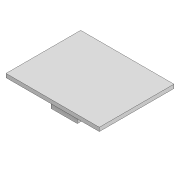
# Autodesk Inventor part: Moving platform
Saved by Autodesk Inventor 2020 (Build 240168000, 168)
## iProperties
Created: 2020-08-18
Part Number: Moving platform
Material: Generic
Document SubType Name: Modeling
Designer: ferrerx
Density: 1 g/cm^3
Appearance: Anodized - Black
Mass: 1.44418 g
Surface Area: 16.2651 cm^2
Volume: 1.44418 cm^3
Author: ferrerx
Autodesk Inventor part; units mm, degrees
ref_plane "YZ Plane" through (0, 0, 0) normal (1, 0, 0) x (0, 1, 0)
ref_plane "XZ Plane" through (0, 0, 0) normal (0, 1, 0) x (-1, 0, 0)
sketch "Sketch1" plane through (0, 0, 0) normal (0, 1, 0) x (-1, 0, 0)
  line L0 (0, 0) -> (25, 0)
  line L1 (25, 0) -> (25, -13.8)
  line L2 (25, -13.8) -> (0, -13.8)
  line L3 (0, -13.8) -> (0, 0)
  dimension "d0" = 25
  dimension "d1" = 13.8
  constraints: 8 end point, 2 parallel, 1 horizontal, 1 perpendicular
  measures "d0" distance of L1.end L2.end
  measures "d1" distance of L2.end L0.start
extrude "Extrusion1" add sketch "Sketch1" along normal blind 4.2
sketch "Sketch2" plane through (0, 0, 0) normal (1, 0, 0) x (0, 0, -1)
  line L0 (0, 0) -> (0, 4.2)
  line L1 (0, 2) -> (13.8, 2)
  line L2 (13.8, 0) -> (13.8, 4.2)
  circle A0 centre (2.4, 2) radius 1.05
  circle A1 centre (11.4, 2) radius 1.05
  line L3 (0, 0) -> (13.8, 0) projected
  line L4 (6.9, 0) -> (6.9, 2.0025)
  line L5 (0, 4.2) -> (13.8, 4.2) projected
  dimension "d4" = 9
  dimension "d7" = 4.5
  dimension "d15" = 2.2
  constraints: 8 end point, 3 point on line, 2 centre point, 1 midpoint, 1 vertical
  measures "d4" distance of A1.centre A0.centre
  measures "d7" distance from line of L4 A0.centre
  measures "d15" distance between parallel lines of L5 L1
extrude "Extrusion2" cut sketch "Sketch2" against normal blind 20 contours A0 L1 | L1 A0 | A1 L1 | L1 A1
sketch "Sketch3" plane through (0, 4.2, 0) normal (0, 1, 0) x (1, 0, 0)
  line L0 (0, 6.9) -> (-25, 6.9)
  line L1 (0, -3.1) -> (-25, -3.1)
  line L2 (-25, -3.1) -> (-25, 16.9)
  line L3 (-25, 16.9) -> (0, 16.9)
  line L4 (0, 16.9) -> (0, -3.1)
  line L5 (0, -3.1) -> (-25, 16.9) construction
  line L6 (-25, -3.1) -> (0, 16.9) construction
  line L7 (-25, 13.8) -> (-25, 0) projected
  line L8 (0, 0) -> (0, 13.8) projected
  line L9 (0, 13.8) -> (-25, 13.8) projected
  point P0 (-12.5, 6.9)
  dimension "d10" = 20
  dimension "d11" = 6.9
  dimension "d12" = 25
  constraints: 14 end point, 5 midpoint, 2 horizontal, 2 parallel, 1 perpendicular
  measures "d10" distance of L3.end L1.start
  measures "d11" distance between parallel lines of L9 L0
  measures "d12" distance of L2.end L3.end
extrude "Extrusion3" add sketch "Sketch3" along normal blind 1
sketch "Sketch4" plane through (0, 5.2, 0) normal (0, 1, 0) x (1, 0, 0)
  circle A0 centre (-21, 12.9) radius 0.25
  line L0 (0, 16.9) -> (-25, 16.9) projected
  line L1 (-25, 16.9) -> (-25, -3.1) projected
  line L2 (-21.25, 12.9) -> (-20.75, 12.9)
  point P0 (0, 0)
  dimension "d16" = 4
  dimension "d17" = 4
  dimension "d18" = 0.5
  constraints: 2 end point, 2 point on circle, 1 centre point, 1 horizontal
  measures "d16" distance from line of L0 A0.centre
  measures "d17" distance from line of L1 A0.centre
  measures "d18" diameter of A0
ref_plane "Work Plane1" through (-21.25, 5.2, -12.9) normal (0, 0, 1) x (1, 0, 0)
sketch "Sketch5" plane through (-21.25, 5.2, -12.9) normal (0, 0, 1) x (1, 0, 0)
  line L0 (-3.75, 0) -> (21.25, 0) projected
  line L1 (0.2469, 0) -> (0.2469, 2)
  line L2 (0.2469, 2) -> (0.9969, 0)
  line L3 (0.9969, 0) -> (0.2469, 0)
  line L4 (21.25, -1) -> (-3.75, -1) projected
  point P0 (21.25, -5.2)
  dimension "d21" = 2
  dimension "d28" = 0.75
  constraints: 6 end point, 1 parallel, 1 point on line, 1 vertical
  measures "d21" distance of L1.start L1.end
  measures "d28" distance of L1.start L2.end
revolve "Revolution1" [suppressed]
pattern_linear "Rectangular Pattern1" [suppressed]
sketch "Sketch6" plane through (0, 0, 0) normal (1, 0, 0) x (0, 0, -1)
  circle A0 centre (2.4, 2) radius 1.05 projected
  circle A1 centre (2.4, 2) radius 1.1
  circle A2 centre (11.4, 2) radius 1.05 projected
  circle A3 centre (11.4, 2) radius 1.1
  point P0 (0, 0)
  dimension "d29" = 2.2
  dimension "d30" = 2.2
  constraints: 2 centre point, 2 coincident
  measures "d29" diameter of A3
  measures "d30" diameter of A1
extrude "Extrusion4" cut sketch "Sketch6" against normal blind 30.5 contours A0 | A1 | A2 | A3
sketch "Sketch7" plane through (0, 5.2, 0) normal (0, 1, 0) x (1, 0, 0)
  line L0 (0, 6.9) -> (-25, 6.9) construction
  line L1 (0, 16.9) -> (-25, 16.9) projected
  line L2 (-13.35, 4.85) -> (-11.65, 4.85)
  line L3 (-11.65, 4.85) -> (-11.65, 8.95)
  line L4 (-11.65, 8.95) -> (-13.35, 8.95)
  line L5 (-13.35, 8.95) -> (-13.35, 4.85)
  line L6 (-13.35, 4.85) -> (-11.65, 8.95) construction
  line L7 (-11.65, 4.85) -> (-13.35, 8.95) construction
  line L8 (0, -3.1) -> (0, 16.9) projected
  point P0 (0, 0)
  point P1 (-12.5, 6.9)
  dimension "d33" = 10
  dimension "d34" = 1.7
  dimension "d35" = 4.1
  dimension "d36" = 11.65
  constraints: 14 end point, 3 midpoint, 2 horizontal, 2 parallel, 1 perpendicular
  measures "d33" distance between parallel lines of L1 L0
  measures "d34" distance of L2.start L2.end
  measures "d35" distance of L2.end L3.end
  measures "d36" distance between parallel lines of L8 L3
extrude "Extrusion5" cut sketch "Sketch7" against normal blind 8.45
sketch "Sketch8" plane through (0, 0, 0) normal (1, 0, 0) x (0, 0, -1)
  circle A0 centre (2.4, 2) radius 1.1 projected
  circle A1 centre (11.4, 2) radius 1.1 projected
  line L0 (2.4, 2) -> (11.4, 2) construction
  circle A2 centre (6.9, 2) radius 1.1
  point P0 (0, 0)
  dimension "d39" = 2.2
  dimension "d40" = 4.5
  constraints: 2 end point, 1 centre point, 1 horizontal, 1 midpoint
  measures "d39" diameter of A2
  measures "d40" distance of L0.start A2.centre
extrude "Extrusion6" cut sketch "Sketch8" against normal blind 31.95 contours A2
sketch "Sketch9" plane through (0, 5.2, 0) normal (0, 1, 0) x (1, 0, 0)
  line L0 (-13.35, 4.85) -> (-13.35, 8.95) projected
  line L1 (-11.65, 4.85) -> (-11.65, 8.95) projected
  line L2 (-13.35, 8.95) -> (-11.65, 8.95)
  line L3 (-11.65, 8.95) -> (-11.65, 4.85)
  line L4 (-11.65, 4.85) -> (-13.35, 4.85)
  line L5 (-13.35, 4.85) -> (-13.35, 8.95)
  point P0 (0, 0)
  constraints: 8 end point, 2 parallel, 1 horizontal, 1 perpendicular
extrude "Extrusion7" add sketch "Sketch9" against normal blind 0.5
sketch "Sketch10" plane through (0, 0, 0) normal (1, 0, 0) x (0, 0, -1)
  line L0 (0, 0) -> (13.8, 0)
  line L1 (13.8, 0) -> (13.8, 4.2)
  line L2 (13.8, 4.2) -> (0, 4.2)
  line L3 (0, 4.2) -> (0, 0)
  line L4 (13.8, 4.2) -> (16.9, 4.2) projected
  line L5 (13.8, 0) -> (13.8, 4.2) projected
  constraints: 8 end point, 2 collinear, 2 parallel, 1 horizontal, 1 perpendicular
extrude "Extrusion8" cut sketch "Sketch10" against normal blind 9
sketch "Sketch11" plane through (-25, 0, -13.8) normal (-1, 0, 0) x (0, 0, 1)
  line L0 (13.8, 0) -> (13.8, 4.2) projected
  line L1 (0, 0) -> (13.8, 0)
  line L2 (13.8, 0) -> (13.8, 4.2)
  line L3 (13.8, 4.2) -> (0, 4.2)
  line L4 (0, 4.2) -> (0, 0)
  line L5 (13.8, 4.2) -> (16.9, 4.2) projected
  constraints: 8 end point, 2 parallel, 1 collinear, 1 horizontal, 1 perpendicular
extrude "Extrusion9" cut sketch "Sketch11" against normal blind 9
body "Solid1"
